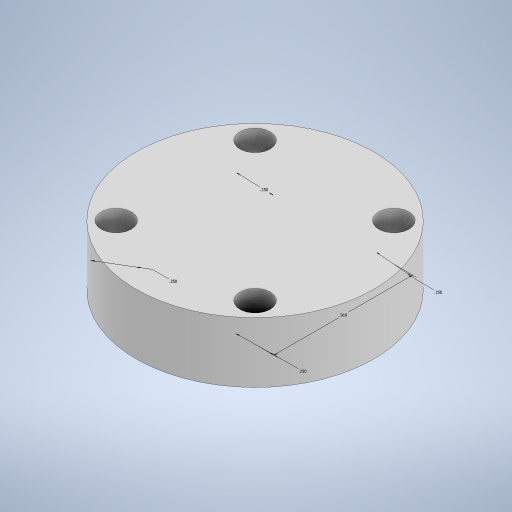
# Autodesk Inventor part: CO-0-01-Planetary1
Saved by Autodesk Inventor 2023 (Build 270158000, 158)
## iProperties
Created: 2023-09-29
Part Number: CO-0-01-Planetary1
Material: Generic
Document SubType Name: Modeling
Designer: thesl
Density: 1 g/cm^3
Appearance: Default
Mass: 12.1515 g
Surface Area: 43.1442 cm^2
Volume: 12.1515 cm^3
Author: thesl
Autodesk Inventor part; units mm, degrees
ref_plane "YZ Plane" through (0, 0, 0) normal (1, 0, 0) x (0, 1, 0)
ref_plane "XZ Plane" through (0, 0, 0) normal (0, 1, 0) x (-1, 0, 0)
ref_plane "XY Plane" through (0, 0, 0) normal (0, 0, 1) x (1, 0, 0)
sketch "Sketch1" plane through (0, 0, 0) normal (0, 1, 0) x (-1, 0, 0)
  circle A0 centre (0, 0) radius 20.0025
  line L0 (-11.6713, 11.6713) -> (11.6713, 11.6713)
  line L1 (11.6713, 11.6713) -> (11.6713, -11.6713)
  line L2 (11.6713, -11.6713) -> (-11.6713, -11.6713)
  line L3 (-11.6713, -11.6713) -> (-11.6713, 11.6713)
  line L4 (-11.6713, 11.6713) -> (11.6713, -11.6713) construction
  line L5 (11.6713, 11.6713) -> (-11.6713, -11.6713) construction
  circle A1 centre (11.6713, -11.6713) radius 1.2446
  circle A2 centre (-11.6713, -11.6713) radius 1.2446
  circle A3 centre (-11.6713, 11.6713) radius 1.2446
  circle A4 centre (11.6713, 11.6713) radius 1.2446
  dimension "d0" = 40.005
  dimension "d1" = 23.3426
  dimension "d2" = 23.3426
  dimension "d3" = 2.4892
  dimension "d4" = 2.4892
  dimension "d5" = 2.4892
  dimension "d6" = 2.4892
  constraints: 12 end point, 5 centre point, 5 coincident, 2 midpoint, 2 parallel, 1 horizontal, 1 perpendicular
  measures "d0" diameter of A0
  measures "d1" distance of L0.start L0.end
  measures "d2" distance of L0.end L1.end
  measures "d3" diameter of A1
  measures "d4" diameter of A2
  measures "d5" diameter of A3
  measures "d6" diameter of A4
extrude "Extrusion1" add sketch "Sketch1" along normal blind 3.81 contours A0 | L0 A4 L1 A1 L2 A2 L3 A3
sketch "Sketch3" plane through (0, 0, 0) normal (0, -1, 0) x (1, 0, 0)
  circle A0 centre (0, 0) radius 1.5875
  dimension "d10" = 3.175
  constraints: 1 centre point, 1 coincident
  measures "d10" diameter of A0
extrude "Extrusion2" cut sketch "Sketch3" against normal blind 6.35
sketch "Sketch5" plane through (0, 3.81, 0) normal (0, 1, 0) x (1, 0, 0)
  circle A0 centre (0, 0) radius 20.0025
  constraints: 1 centre point, 1 coincident
sketch "Sketch6" plane through (0, 3.81, 0) normal (0, 1, 0) x (1, 0, 0)
  line L0 (-11.6713, 11.6713) -> (11.6713, 11.6713)
  line L1 (11.6713, 11.6713) -> (11.6713, -11.6713)
  line L2 (11.6713, -11.6713) -> (-11.6713, -11.6713)
  line L3 (-11.6713, -11.6713) -> (-11.6713, 11.6713)
  circle A0 centre (0, 0) radius 1.5875 projected
  line L4 (-11.6713, 11.6713) -> (11.6713, -11.6713) construction
  line L5 (11.6713, 11.6713) -> (-11.6713, -11.6713) construction
  circle A1 centre (-11.6713, 11.6713) radius 3.175
  circle A2 centre (11.6713, 11.6713) radius 3.175
  circle A3 centre (11.6713, -11.6713) radius 3.175
  circle A4 centre (-11.6713, -11.6713) radius 1.2446 projected
  circle A5 centre (-11.6713, -11.6713) radius 3.175
  dimension "d13" = 23.3426
  dimension "d14" = 6.35
  dimension "d15" = 6.35
  dimension "d16" = 6.35
  dimension "d17" = 6.35
  constraints: 12 end point, 4 centre point, 4 coincident, 2 midpoint, 2 parallel, 1 horizontal, 1 perpendicular
  measures "d13" distance of L0.end L1.end
  measures "d14" diameter of A1
  measures "d15" diameter of A2
  measures "d16" diameter of A3
  measures "d17" diameter of A5
extrude "Extrusion3" add sketch "Sketch5" along normal blind 6.35
sketch "Sketch7" plane through (0, 10.16, 0) normal (0, 1, 0) x (1, 0, 0)
  line L0 (-11.6713, -11.6713) -> (11.6713, -11.6713)
  line L1 (11.6713, -11.6713) -> (11.6713, 11.6713)
  line L2 (11.6713, 11.6713) -> (-11.6713, 11.6713)
  line L3 (-11.6713, 11.6713) -> (-11.6713, -11.6713)
  circle A0 centre (0, 0) radius 1.5875 projected
  line L4 (-11.6713, -11.6713) -> (11.6713, 11.6713) construction
  line L5 (11.6713, -11.6713) -> (-11.6713, 11.6713) construction
  circle A1 centre (-11.6713, 11.6713) radius 1.2446 projected
  circle A2 centre (-11.6713, 11.6713) radius 2.54
  circle A3 centre (11.6713, 11.6713) radius 1.2446 projected
  circle A4 centre (11.6713, 11.6713) radius 2.54
  circle A5 centre (11.6713, -11.6713) radius 1.2446 projected
  circle A6 centre (11.6713, -11.6713) radius 2.54
  circle A7 centre (-11.6713, -11.6713) radius 1.2446 projected
  circle A8 centre (-11.6713, -11.6713) radius 2.54
  dimension "d20" = 23.3426
  dimension "d21" = 23.3426
  dimension "d22" = 5.08
  dimension "d23" = 5.08
  dimension "d24" = 5.08
  dimension "d25" = 5.08
  constraints: 12 end point, 4 centre point, 4 coincident, 2 midpoint, 2 parallel, 1 horizontal, 1 perpendicular
  measures "d20" distance of L0.start L0.end
  measures "d21" distance of L1.end L0.end
  measures "d22" diameter of A2
  measures "d23" diameter of A4
  measures "d24" diameter of A6
  measures "d25" diameter of A8
extrude "Extrusion4" cut sketch "Sketch7" against normal blind 6.35 contours L3 A7 L0 | L0 A7 L3 | A7 L3 A8 L0 | L0 A8 L3 A7 | A6 L1 A5 L0 | L0 A5 L1 A6 | A2 L2 A1 L3 | L3 A1 L2 A2 | A5 L1 L0 | L0 L1 A5 | A1 L2 L3 | L3 L2 A1 | A4 L2 A3 L1 | L1 A3 L2 A4 | A3 L2 L1 | L1 L2 A3
body "Solid1"
